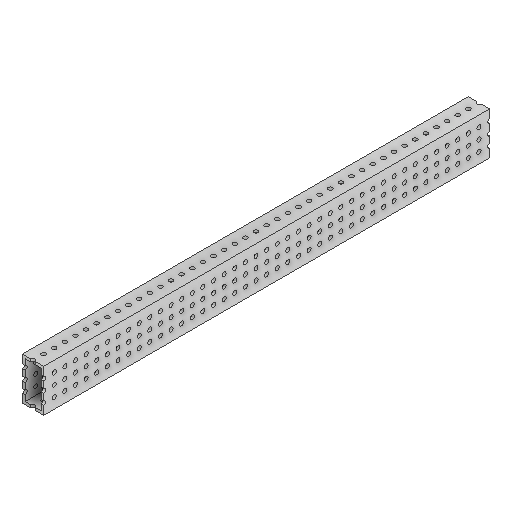
# Autodesk Inventor part: Foja - Base Chassi
Saved by Autodesk Inventor 2025.3 (Build 293356000, 356)
## iProperties
Created: 2026-05-13
Part Number: Foja - Base Chassi
Material: Genérico
Document SubType Name: Modeling
Designer: djair.oliveira
Density: 1 g/cm^3
Appearance: Padrão
Author: djair.oliveira
Autodesk Inventor part; units mm, degrees
ref_plane "YZ Plane" through (0, 0, 0) normal (1, 0, 0) x (0, 1, 0)
ref_plane "XZ Plane" through (0, 0, 0) normal (0, 1, 0) x (-1, 0, 0)
ref_plane "XY Plane" through (0, 0, 0) normal (0, 0, 1) x (1, 0, 0)
sketch "Esboço1" plane through (0, 0, 0) normal (0, 0, 1) x (1, 0, 0)
  line L0 (12.7, -25.4) -> (-12.7, -25.4)
  line L1 (-12.7, -25.4) -> (-12.7, 25.4)
  line L2 (-12.7, 25.4) -> (12.7, 25.4)
  line L3 (12.7, 25.4) -> (12.7, -25.4)
  line L4 (12.7, -25.4) -> (-12.7, 25.4) construction
  line L5 (-12.7, -25.4) -> (12.7, 25.4) construction
  line L6 (9.525, -22.225) -> (-9.525, -22.225)
  line L7 (-9.525, -22.225) -> (-9.525, 22.225)
  line L8 (-9.525, 22.225) -> (9.525, 22.225)
  line L9 (9.525, 22.225) -> (9.525, -22.225)
  line L10 (9.525, -22.225) -> (-9.525, 22.225) construction
  line L11 (-9.525, -22.225) -> (9.525, 22.225) construction
  point P0 (0, 0)
  dimension "d1" = 3.175
  dimension "d2" = 3.175
  dimension "d3" = 25.4
  dimension "d4" = 50.8
  constraints: 24 end point, 4 midpoint, 4 parallel, 2 horizontal, 2 perpendicular
  measures "d1" distance between parallel lines of L1 L7
  measures "d2" distance between parallel lines of L2 L8
  measures "d3" distance of L1.end L2.end
  measures "d4" distance of L2.end L0.start
extrude "Extrusão1" add sketch "Esboço1" along normal blind 533.4
sketch "Esboço2" plane through (-12.7, 25.4, 0) normal (0, 1, 0) x (1, 0, 0)
  circle A0 centre (12.7, -266.7) radius 2.5
  line L0 (0, 0) -> (0, -533.4) projected
  line L1 (25.4, -533.4) -> (0, -533.4) projected
  line L2 (25.4, 0) -> (0, 0) projected
  circle A1 centre (12.7, -279.4) radius 2.5
  circle A2 centre (12.7, -254) radius 2.5
  circle A3 centre (12.7, -292.1) radius 2.5
  circle A4 centre (12.7, -241.3) radius 2.5
  circle A5 centre (12.7, -304.8) radius 2.5
  circle A6 centre (12.7, -228.6) radius 2.5
  circle A7 centre (12.7, -317.5) radius 2.5
  circle A8 centre (12.7, -215.9) radius 2.5
  circle A9 centre (12.7, -330.2) radius 2.5
  circle A10 centre (12.7, -203.2) radius 2.5
  circle A11 centre (12.7, -342.9) radius 2.5
  circle A12 centre (12.7, -190.5) radius 2.5
  circle A13 centre (12.7, -355.6) radius 2.5
  circle A14 centre (12.7, -177.8) radius 2.5
  circle A15 centre (12.7, -368.3) radius 2.5
  circle A16 centre (12.7, -165.1) radius 2.5
  circle A17 centre (12.7, -381) radius 2.5
  circle A18 centre (12.7, -152.4) radius 2.5
  circle A19 centre (12.7, -393.7) radius 2.5
  circle A20 centre (12.7, -139.7) radius 2.5
  circle A21 centre (12.7, -406.4) radius 2.5
  circle A22 centre (12.7, -127) radius 2.5
  circle A23 centre (12.7, -419.1) radius 2.5
  circle A24 centre (12.7, -114.3) radius 2.5
  circle A25 centre (12.7, -431.8) radius 2.5
  circle A26 centre (12.7, -101.6) radius 2.5
  circle A27 centre (12.7, -444.5) radius 2.5
  circle A28 centre (12.7, -88.9) radius 2.5
  circle A29 centre (12.7, -457.2) radius 2.5
  circle A30 centre (12.7, -76.2) radius 2.5
  circle A31 centre (12.7, -469.9) radius 2.5
  circle A32 centre (12.7, -63.5) radius 2.5
  circle A33 centre (12.7, -482.6) radius 2.5
  circle A34 centre (12.7, -50.8) radius 2.5
  circle A35 centre (12.7, -495.3) radius 2.5
  circle A36 centre (12.7, -38.1) radius 2.5
  circle A37 centre (12.7, -508) radius 2.5
  circle A38 centre (12.7, -25.4) radius 2.5
  circle A39 centre (12.7, -520.7) radius 2.5
  circle A40 centre (12.7, -12.7) radius 2.5
  circle A41 centre (12.7, -533.4) radius 2.5
  circle A42 centre (12.7, 0) radius 2.5
  point P0 (12.7, 0)
  point P1 (12.7, -533.4)
  point P2 (12.7, 0)
  point P3 (12.7, 0)
  dimension "d7" = 5
  dimension "d8" = 12.7
  dimension "d9" = 533.4
  dimension "d10" = 266.7
  dimension "d13" = 12.7
  constraints: 43 centre point, 3 midpoint, 1 vertical, 84 other
  measures "d7" diameter of A0
  measures "d8" distance from line of L0 A0.centre
  measures "d9" distance of point (12.7, -533.4) point (12.7, 0)
  measures "d10" distance of point (12.7, 0) A0.centre
  measures "d13" distance of A0.centre A1.centre
extrude "Extrusão2" cut sketch "Esboço2" against normal up to surface (50.8 mm away)
sketch "Esboço3" plane through (12.7, -25.4, 0) normal (1, 0, 0) x (0, 0, -1)
  circle A0 centre (-266.7, 38.1) radius 2.5
  circle A1 centre (-266.7, 25.4) radius 2.5
  circle A2 centre (-266.7, 12.7) radius 2.5
  line L0 (0, 50.8) -> (-533.4, 50.8) projected
  line L1 (-266.7, 50.8) -> (-266.7, 0)
  line L2 (0, 0) -> (-533.4, 0) projected
  circle A3 centre (-279.4, 38.1) radius 2.5
  circle A4 centre (-279.4, 25.4) radius 2.5
  circle A5 centre (-279.4, 12.7) radius 2.5
  circle A6 centre (-254, 38.1) radius 2.5
  circle A7 centre (-254, 25.4) radius 2.5
  circle A8 centre (-254, 12.7) radius 2.5
  circle A9 centre (-292.1, 38.1) radius 2.5
  circle A10 centre (-292.1, 25.4) radius 2.5
  circle A11 centre (-292.1, 12.7) radius 2.5
  circle A12 centre (-241.3, 38.1) radius 2.5
  circle A13 centre (-241.3, 25.4) radius 2.5
  circle A14 centre (-241.3, 12.7) radius 2.5
  circle A15 centre (-304.8, 38.1) radius 2.5
  circle A16 centre (-304.8, 25.4) radius 2.5
  circle A17 centre (-304.8, 12.7) radius 2.5
  circle A18 centre (-228.6, 38.1) radius 2.5
  circle A19 centre (-228.6, 25.4) radius 2.5
  circle A20 centre (-228.6, 12.7) radius 2.5
  circle A21 centre (-317.5, 38.1) radius 2.5
  circle A22 centre (-317.5, 25.4) radius 2.5
  circle A23 centre (-317.5, 12.7) radius 2.5
  circle A24 centre (-215.9, 38.1) radius 2.5
  circle A25 centre (-215.9, 25.4) radius 2.5
  circle A26 centre (-215.9, 12.7) radius 2.5
  circle A27 centre (-330.2, 38.1) radius 2.5
  circle A28 centre (-330.2, 25.4) radius 2.5
  circle A29 centre (-330.2, 12.7) radius 2.5
  circle A30 centre (-203.2, 38.1) radius 2.5
  circle A31 centre (-203.2, 25.4) radius 2.5
  circle A32 centre (-203.2, 12.7) radius 2.5
  circle A33 centre (-342.9, 38.1) radius 2.5
  circle A34 centre (-342.9, 25.4) radius 2.5
  circle A35 centre (-342.9, 12.7) radius 2.5
  circle A36 centre (-190.5, 38.1) radius 2.5
  circle A37 centre (-190.5, 25.4) radius 2.5
  circle A38 centre (-190.5, 12.7) radius 2.5
  circle A39 centre (-355.6, 38.1) radius 2.5
  circle A40 centre (-355.6, 25.4) radius 2.5
  circle A41 centre (-355.6, 12.7) radius 2.5
  circle A42 centre (-177.8, 38.1) radius 2.5
  circle A43 centre (-177.8, 25.4) radius 2.5
  circle A44 centre (-177.8, 12.7) radius 2.5
  circle A45 centre (-368.3, 38.1) radius 2.5
  circle A46 centre (-368.3, 25.4) radius 2.5
  circle A47 centre (-368.3, 12.7) radius 2.5
  circle A48 centre (-165.1, 38.1) radius 2.5
  circle A49 centre (-165.1, 25.4) radius 2.5
  circle A50 centre (-165.1, 12.7) radius 2.5
  circle A51 centre (-381, 38.1) radius 2.5
  circle A52 centre (-381, 25.4) radius 2.5
  circle A53 centre (-381, 12.7) radius 2.5
  circle A54 centre (-152.4, 38.1) radius 2.5
  circle A55 centre (-152.4, 25.4) radius 2.5
  circle A56 centre (-152.4, 12.7) radius 2.5
  circle A57 centre (-393.7, 38.1) radius 2.5
  circle A58 centre (-393.7, 25.4) radius 2.5
  circle A59 centre (-393.7, 12.7) radius 2.5
  circle A60 centre (-139.7, 38.1) radius 2.5
  circle A61 centre (-139.7, 25.4) radius 2.5
  circle A62 centre (-139.7, 12.7) radius 2.5
  circle A63 centre (-406.4, 38.1) radius 2.5
  circle A64 centre (-406.4, 25.4) radius 2.5
  circle A65 centre (-406.4, 12.7) radius 2.5
  circle A66 centre (-127, 38.1) radius 2.5
  circle A67 centre (-127, 25.4) radius 2.5
  circle A68 centre (-127, 12.7) radius 2.5
  circle A69 centre (-419.1, 38.1) radius 2.5
  circle A70 centre (-419.1, 25.4) radius 2.5
  circle A71 centre (-419.1, 12.7) radius 2.5
  circle A72 centre (-114.3, 38.1) radius 2.5
  circle A73 centre (-114.3, 25.4) radius 2.5
  circle A74 centre (-114.3, 12.7) radius 2.5
  circle A75 centre (-431.8, 38.1) radius 2.5
  circle A76 centre (-431.8, 25.4) radius 2.5
  circle A77 centre (-431.8, 12.7) radius 2.5
  circle A78 centre (-101.6, 38.1) radius 2.5
  circle A79 centre (-101.6, 25.4) radius 2.5
  circle A80 centre (-101.6, 12.7) radius 2.5
  circle A81 centre (-444.5, 38.1) radius 2.5
  circle A82 centre (-444.5, 25.4) radius 2.5
  circle A83 centre (-444.5, 12.7) radius 2.5
  circle A84 centre (-88.9, 38.1) radius 2.5
  circle A85 centre (-88.9, 25.4) radius 2.5
  circle A86 centre (-88.9, 12.7) radius 2.5
  circle A87 centre (-457.2, 38.1) radius 2.5
  circle A88 centre (-457.2, 25.4) radius 2.5
  circle A89 centre (-457.2, 12.7) radius 2.5
  circle A90 centre (-76.2, 38.1) radius 2.5
  circle A91 centre (-76.2, 25.4) radius 2.5
  circle A92 centre (-76.2, 12.7) radius 2.5
  circle A93 centre (-469.9, 38.1) radius 2.5
  circle A94 centre (-469.9, 25.4) radius 2.5
  circle A95 centre (-469.9, 12.7) radius 2.5
  circle A96 centre (-63.5, 38.1) radius 2.5
  circle A97 centre (-63.5, 25.4) radius 2.5
  circle A98 centre (-63.5, 12.7) radius 2.5
  circle A99 centre (-482.6, 38.1) radius 2.5
  circle A100 centre (-482.6, 25.4) radius 2.5
  circle A101 centre (-482.6, 12.7) radius 2.5
  circle A102 centre (-50.8, 38.1) radius 2.5
  circle A103 centre (-50.8, 25.4) radius 2.5
  circle A104 centre (-50.8, 12.7) radius 2.5
  circle A105 centre (-495.3, 38.1) radius 2.5
  circle A106 centre (-495.3, 25.4) radius 2.5
  circle A107 centre (-495.3, 12.7) radius 2.5
  circle A108 centre (-38.1, 38.1) radius 2.5
  circle A109 centre (-38.1, 25.4) radius 2.5
  circle A110 centre (-38.1, 12.7) radius 2.5
  circle A111 centre (-508, 38.1) radius 2.5
  circle A112 centre (-508, 25.4) radius 2.5
  circle A113 centre (-508, 12.7) radius 2.5
  circle A114 centre (-25.4, 38.1) radius 2.5
  circle A115 centre (-25.4, 25.4) radius 2.5
  circle A116 centre (-25.4, 12.7) radius 2.5
  circle A117 centre (-520.7, 38.1) radius 2.5
  circle A118 centre (-520.7, 25.4) radius 2.5
  circle A119 centre (-520.7, 12.7) radius 2.5
  circle A120 centre (-12.7, 38.1) radius 2.5
  circle A121 centre (-12.7, 25.4) radius 2.5
  circle A122 centre (-12.7, 12.7) radius 2.5
  circle A123 centre (-533.4, 38.1) radius 2.5
  circle A124 centre (-533.4, 25.4) radius 2.5
  circle A125 centre (-533.4, 12.7) radius 2.5
  circle A126 centre (0, 38.1) radius 2.5
  circle A127 centre (0, 25.4) radius 2.5
  circle A128 centre (0, 12.7) radius 2.5
  point P0 (0, 25.4)
  dimension "d20" = 5
  dimension "d21" = 25.4
  dimension "d22" = 12.7
  dimension "d23" = 12.7
  dimension "d26" = 12.7
  constraints: 129 centre point, 2 end point, 2 equal radius, 2 midpoint, 2 vertical alignment, 1 horizontal, 1 point on line, 252 other
  measures "d20" diameter of A1
  measures "d21" distance from line of L0 A1.centre
  measures "d22" distance of A0.centre A1.centre
  measures "d23" distance of A2.centre A1.centre
  measures "d26" distance of A0.centre A3.centre
extrude "Extrusão3" cut sketch "Esboço3" against normal up to surface (25.4 mm away)
equation "\"d2\" = d1"
equation "\"d10\" = 0.5 * d9"
equation "\"d23\" = d22"
